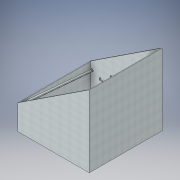
# Autodesk Inventor part: caixa
Saved by Autodesk Inventor 2019.4 (Build 234330000, 330)
## iProperties
Created: 2020-04-10
Part Number: caixa
Material: Polipropileno
Document SubType Name: Modeling
Designer: lucas
Density: 0.899 g/cm^3
Appearance: Madeira - Pintada de branco
Author: lucas
Autodesk Inventor part; units mm, degrees
ref_plane "YZ Plane" through (0, 0, 0) normal (1, 0, 0) x (0, 1, 0)
ref_plane "XZ Plane" through (0, 0, 0) normal (0, 1, 0) x (-1, 0, 0)
sketch "Esboço1" plane through (0, 0, 0) normal (0, 0, 1) x (1, 0, 0)
  line L0 (0, 0) -> (1000, 0)
  line L1 (1000, 0) -> (1000, 1000)
  line L2 (0, 0) -> (0, 350)
  line L3 (990, 1000) -> (990, 10)
  line L4 (990, 10) -> (10, 10)
  line L5 (10, 10) -> (10, 350)
  line L6 (0, 350) -> (10, 350)
  line L7 (990, 1000) -> (1000, 1000)
  line L8 (0, 350) -> (10, 350)
  line L9 (990, 1000) -> (1000, 1000)
  dimension "d6" = 1000
  dimension "d7" = 1000
  dimension "d8" = 350
  dimension "d10" = 10
  constraints: 20 end point, 3 parallel, 3 perpendicular, 1 horizontal, 1 vertical, 2 other
  measures "d6" distance of L0.start L0.end
  measures "d7" distance of L0.end L1.end
  measures "d8" distance of L0.start L2.end
  measures "d10" distance between parallel lines of L1 L3
extrude "Extrusão1" add sketch "Esboço1" along normal blind 1000
sketch "Esboço2" plane through (0, 0, 1000) normal (0, 0, 1) x (1, 0, 0)
  line L0 (10, 10) -> (10, 350) projected
  line L1 (0, 350) -> (0, 0) projected
  line L2 (1000, 1000) -> (990, 1000) projected
  line L3 (0, 350) -> (990, 1000)
  line L4 (0, 0) -> (1000, 0) projected
  line L5 (1000, 0) -> (1000, 1000) projected
  line L6 (0, 350) -> (0, 0)
  line L7 (1000, 0) -> (1000, 1000)
  line L8 (990, 1000) -> (1000, 1000)
  constraints: 8 end point, 2 collinear, 1 vertical
extrude "Extrusão2" add sketch "Esboço2" along normal blind 10
sketch "Esboço3" plane through (0, 0, 0) normal (0, 0, -1) x (-1, 0, 0)
  line L0 (-10, 350) -> (0, 350) projected
  line L1 (-1000, 1000) -> (-990, 1000) projected
  line L2 (0, 350) -> (-990, 1000)
  line L3 (-990, 1000) -> (-1000, 1000)
  line L4 (-1000, 1000) -> (-1000, 0)
  line L5 (0, 0) -> (-1000, 0) projected
  line L6 (-1000, 0) -> (0, 0)
  line L7 (0, 0) -> (0, 350)
  constraints: 10 end point, 2 collinear, 2 perpendicular
extrude "Extrusão3" add sketch "Esboço3" along normal blind 10
sketch "Esboço4" plane through (10, 10, 1000) normal (1, 0, 0) x (0, 0, -1)
  line L0 (1000, 990) -> (1000, 0) projected
  line L1 (1000, 232.5113) -> (0, 320)
  line L2 (0, 0) -> (0, 340) projected
  line L3 (0, 340) -> (-10, 340) projected
  line L4 (1000, 242.5495) -> (0, 330.0382)
  line L5 (1000, 232.5113) -> (1000, 242.5495)
  line L6 (1000, 0) -> (1000, 340) projected
  line L7 (0, 330.0382) -> (0, 320)
  point P0 (1000, -10)
  dimension "d11" = 85
  dimension "d13" = 20
  dimension "d14" = 10
  constraints: 8 end point, 4 point on line, 1 collinear, 1 parallel
  measures "d11" angle of L2 L1
  measures "d13" distance from line of L3 L1.end
  measures "d14" distance between parallel lines of L1 L4
extrude "Extrusão4" add sketch "Esboço4" along normal blind 30
sketch "Esboço5" plane through (40, 10, 1000) normal (1, 0, 0) x (0, 0, -1)
  line L0 (1000, 232.5113) -> (0, 320) projected
  line L1 (1000, 232.5113) -> (0, 320)
  line L2 (0, 336.0611) -> (1000, 248.5725)
  line L3 (1000, 242.5495) -> (1000, 340) projected
  line L4 (1000, 248.5725) -> (1000, 242.5495)
  line L5 (0, 336.0611) -> (0, 320)
  line L6 (0, 330.0382) -> (0, 340) projected
  line L7 (1000, 0) -> (1000, 232.5113) projected
  line L8 (1000, 232.5113) -> (0, 320)
  line L9 (0, 330.0382) -> (1000, 242.5495) projected
  point P0 (1000, -10)
  dimension "d18" = 6
  constraints: 10 end point, 4 collinear, 1 point on line
  measures "d18" distance between parallel lines of L9 L2
extrude "Extrusão5" add sketch "Esboço5" along normal blind 10
sketch "Esboço6" plane through (0, 0, 0) normal (0, 0, 1) x (1, 0, 0)
  line L0 (10, 252.5495) -> (10, 350) projected
  line L1 (10, 252.5495) -> (40, 252.5495)
  line L2 (40, 252.5495) -> (40, 273.6954)
  line L3 (40, 273.6954) -> (10, 273.6954)
  line L4 (10, 273.6954) -> (10, 252.5495)
  point P0 (0, 0)
  constraints: 8 end point, 2 parallel, 1 horizontal, 1 perpendicular
extrude "Extrusão6" cut sketch "Esboço6" against normal blind 10
sketch "Esboço7" plane through (0, 0, 0) normal (0, 0, 1) x (1, 0, 0)
  line L0 (0, 350) -> (990, 1000) projected
  line L1 (591.5971, 523.0033) -> (591.5971, 493.0033)
  line L2 (591.5971, 493.0033) -> (793.5971, 493.0033)
  line L3 (793.5971, 493.0033) -> (793.5971, 553.0033)
  line L4 (793.5971, 553.0033) -> (783.5971, 553.0033)
  line L5 (783.5971, 553.0033) -> (783.5971, 503.0033)
  line L6 (783.5971, 503.0033) -> (601.5971, 503.0033)
  line L7 (601.5971, 503.0033) -> (601.5971, 523.0033)
  line L8 (601.5971, 523.0033) -> (591.5971, 523.0033)
  line L9 (0, 0) -> (0, 350) projected
  line L10 (441.0647, 423.0033) -> (441.0647, 393.0033)
  line L11 (441.0647, 393.0033) -> (643.0647, 393.0033)
  line L12 (643.0647, 393.0033) -> (643.0647, 453.0033)
  line L13 (643.0647, 453.0033) -> (633.0647, 453.0033)
  line L14 (633.0647, 453.0033) -> (633.0647, 403.0033)
  line L15 (633.0647, 403.0033) -> (451.0647, 403.0033)
  line L16 (451.0647, 403.0033) -> (451.0647, 423.0033)
  line L17 (451.0647, 423.0033) -> (441.0647, 423.0033)
  line L18 (290.5324, 323.0033) -> (290.5324, 293.0033)
  line L19 (290.5324, 293.0033) -> (492.5324, 293.0033)
  line L20 (492.5324, 293.0033) -> (492.5324, 353.0033)
  line L21 (492.5324, 353.0033) -> (482.5324, 353.0033)
  line L22 (482.5324, 353.0033) -> (482.5324, 303.0033)
  line L23 (482.5324, 303.0033) -> (300.5324, 303.0033)
  line L24 (300.5324, 303.0033) -> (300.5324, 323.0033)
  line L25 (300.5324, 323.0033) -> (290.5324, 323.0033)
  line L26 (140, 223.0033) -> (140, 193.0033)
  line L27 (140, 193.0033) -> (342, 193.0033)
  line L28 (342, 193.0033) -> (342, 253.0033)
  line L29 (342, 253.0033) -> (332, 253.0033)
  line L30 (332, 253.0033) -> (332, 203.0033)
  line L31 (332, 203.0033) -> (150, 203.0033)
  line L32 (150, 203.0033) -> (150, 223.0033)
  line L33 (150, 223.0033) -> (140, 223.0033)
  line L34 (0, 100) -> (1000, 764.309)
  line L35 (1000, 1000) -> (1000, 0) projected
  line L36 (742.1294, 623.0033) -> (742.1294, 593.0033)
  line L37 (742.1294, 593.0033) -> (944.1294, 593.0033)
  line L38 (944.1294, 593.0033) -> (944.1294, 653.0033)
  line L39 (944.1294, 653.0033) -> (934.1294, 653.0033)
  line L40 (934.1294, 653.0033) -> (934.1294, 603.0033)
  line L41 (934.1294, 603.0033) -> (752.1294, 603.0033)
  line L42 (752.1294, 603.0033) -> (752.1294, 623.0033)
  line L43 (752.1294, 623.0033) -> (742.1294, 623.0033)
  dimension "d23" = 202
  dimension "d24" = 10
  dimension "d25" = 10
  dimension "d26" = 10
  dimension "d27" = 30
  dimension "d28" = 60
  dimension "d35" = 202
  dimension "d36" = 10
  dimension "d37" = 10
  dimension "d38" = 10
  dimension "d39" = 30
  dimension "d40" = 60
  dimension "d41" = 202
  dimension "d42" = 10
  dimension "d43" = 10
  dimension "d44" = 10
  dimension "d45" = 30
  dimension "d46" = 60
  dimension "d47" = 202
  dimension "d48" = 10
  dimension "d49" = 10
  dimension "d50" = 10
  dimension "d51" = 30
  dimension "d52" = 60
  dimension "d53" = 100
  dimension "d54" = 202
  dimension "d55" = 10
  dimension "d56" = 10
  dimension "d57" = 10
  dimension "d58" = 30
  dimension "d59" = 60
  dimension "d60" = 90
  dimension "d61" = 90
  dimension "d62" = 90
  dimension "d63" = 90
  dimension "d64" = 764.309
  dimension "d65" = 140
  constraints: 82 end point, 30 perpendicular, 7 point on line, 5 horizontal, 5 vertical
  measures "d23" distance of L1.end L2.end
  measures "d24" distance between parallel lines of L3 L5
  measures "d25" distance between parallel lines of L7 L1
  measures "d26" distance between parallel lines of L2 L6
  measures "d27" distance between parallel lines of L2 L8
  measures "d28" distance between parallel lines of L2 L4
  measures "d35" distance of L10.end L11.end
  measures "d36" distance between parallel lines of L12 L14
  measures "d37" distance between parallel lines of L16 L10
  measures "d38" distance between parallel lines of L11 L15
  measures "d39" distance between parallel lines of L11 L17
  measures "d40" distance between parallel lines of L11 L13
  measures "d41" distance of L18.end L19.end
  measures "d42" distance between parallel lines of L20 L22
  measures "d43" distance between parallel lines of L24 L18
  measures "d44" distance between parallel lines of L19 L23
  measures "d45" distance between parallel lines of L19 L25
  measures "d46" distance between parallel lines of L19 L21
  measures "d47" distance of L26.end L28.start
  measures "d48" distance between parallel lines of L28 L30
  measures "d49" distance between parallel lines of L32 L26
  measures "d50" distance between parallel lines of L27 L31
  measures "d51" distance between parallel lines of L27 L33
  measures "d52" distance between parallel lines of L27 L29
  measures "d53" distance of L9.start L34.start
  measures "d54" distance of L36.end L37.end
  measures "d55" distance between parallel lines of L38 L40
  measures "d56" distance between parallel lines of L42 L36
  measures "d57" distance between parallel lines of L37 L41
  measures "d58" distance between parallel lines of L37 L43
  measures "d59" distance between parallel lines of L37 L39
  measures "d60" distance between parallel lines of L31 L19
  measures "d61" distance between parallel lines of L23 L11
  measures "d62" distance between parallel lines of L15 L2
  measures "d63" distance between parallel lines of L6 L37
  measures "d64" distance of L35.end L34.end
  measures "d65" distance between parallel lines of L9 L26
extrude "Extrusão7" add sketch "Esboço7" along normal blind 10
ref_plane "Plano de trabalho1" through (0, 0, 500) normal (0, 0, 1) x (1, 0, 0)
mirror "Espelhamento1" about plane through (0, 0, 500) normal (0, 0, 1) of "Extrusão7"
sketch "Esboço8" plane through (0, 0, 0) normal (0, 0, 1) x (1, 0, 0)
  circle A0 centre (41.0461, 30) radius 15.525
  line L0 (990, 10) -> (10, 10) projected
  point P0 (0, 0)
  dimension "d68" = 31.05
  dimension "d69" = 20
  constraints: 1 centre point
  measures "d68" diameter of A0
  measures "d69" distance from line of L0 A0.centre
extrude "Extrusão8" cut sketch "Esboço8" against normal blind 10
